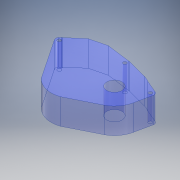
# Autodesk Inventor part: body droit
Saved by Autodesk Inventor 2018.1 (Build 221171000, 171)
## iProperties
Created: 2022-07-20
Part Number: body droit
Material: Generic
Document SubType Name: Modeling
Designer: mouta
Density: 1 g/cm^3
Appearance: Default
Author: mouta
Autodesk Inventor part; units mm, degrees
ref_plane "YZ Plane" through (0, 0, 0) normal (1, 0, 0) x (0, 1, 0)
ref_plane "XZ Plane" through (0, 0, 0) normal (0, 1, 0) x (-1, 0, 0)
ref_plane "XY Plane" through (0, 0, 0) normal (0, 0, 1) x (1, 0, 0)
sketch "Sketch1" plane through (0, 0, 0) normal (0, 0, 1) x (1, 0, 0)
  circle A0 centre (0, 0) radius 3
  circle A1 centre (149.4, 0) radius 3
  circle A2 centre (85.7991, 21.6971) radius 3
  circle A3 centre (110.2989, -19.8991) radius 12.5
  arc A4 (87.814, 27.3487) -> (83.7842, 27.3487) centre (85.7991, 21.6971) ccw
  arc A5 (154.885, -2.4321) -> (151.3594, 5.6711) centre (149.4, 0) ccw
  arc A6 (-0.9713, 5.9209) -> (-1.9594, -5.6711) centre (0, 0) ccw
  line L0 (-1.9594, 5.6711) -> (-0.9713, 5.9209)
  line L1 (87.814, 27.3487) -> (120.8026, 18.6971)
  line L2 (131.5219, 14.0064) -> (151.3594, 5.6711)
  line L3 (155.4, 0) -> (149.4311, -28.1861)
  arc A7 (131.5219, 14.0064) -> (120.0887, 18.8843) centre (110.2989, -19.8991) ccw
  line L4 (21.1662, 25.9822) -> (47.4365, 32.6255)
  line L5 (-4.9033, 3.458) -> (21.1662, 25.9822)
  line L6 (85.7991, 27.6971) -> (47.4365, 32.6255)
  line L7 (0, 0) -> (2.9084, 0.7355)
  line L8 (82.8907, 20.9616) -> (85.7991, 21.6971)
  arc A8 (125.9738, -56.7) -> (149.4311, -28.1861) centre (110.2989, -19.8991) ccw
  line L9 (80.7723, -79.2884) -> (129.3991, -55.0443)
  line L10 (-4.37, -4.1113) -> (37.9799, -67.1663)
  arc A9 (88.5511, 22.8914) -> (86.7834, 21.946) centre (110.2989, -19.8991) ccw
  arc A10 (154.9491, -2.282) -> (150.7621, 5.922) centre (110.2989, -19.8991) ccw
  arc A11 (33.9775, -61.2072) -> (80.7723, -79.2884) centre (68.0362, -42.6558) ccw
  point P0 (111.3369, -59.8857)
  dimension "d3" = 6
  dimension "d5" = 6
  dimension "d15" = 6
  dimension "d18" = 25
  dimension "d19" = 12
  dimension "d20" = 12
  dimension "d21" = 12
  constraints: 29 point on circle, 22 end point, 11 centre point, 5 coincident, 5 point on line, 2 parallel, 1 tangent, 3 other
  measures "d5" diameter of A1
  measures "d15" diameter of A2
  measures "d18" diameter of A3
  measures "d19" diameter of A4
  measures "d20" diameter of A5
  measures "d21" diameter of A6
extrude "Extrusion2" add sketch "Sketch1" along normal blind 42 contours L1 A7 L2 A10 L3 A8 L9 A11 L10 A6 L5 L4 L6 A4 | L2 A5 L3 A10
body "Solid2"
